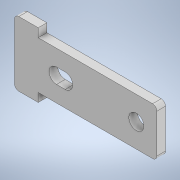
# Autodesk Inventor part: Крепеж
Saved by Autodesk Inventor 2021 (Build 250183000, 183)
## iProperties
Created: 2022-07-08
Part Number: Крепеж
Material: Типовые
Document SubType Name: Modeling
Designer: zvi20
Density: 1 g/cm^3
Appearance: По умолчанию
Author: zvi20
Autodesk Inventor part; units mm, degrees
ref_plane "YZ Plane" through (0, 0, 0) normal (1, 0, 0) x (0, 1, 0)
ref_plane "XZ Plane" through (0, 0, 0) normal (0, 1, 0) x (-1, 0, 0)
ref_plane "XY Plane" through (0, 0, 0) normal (0, 0, 1) x (1, 0, 0)
sketch "Эскиз1" plane through (0, 0, 0) normal (0, 0, 1) x (1, 0, 0)
  line L0 (-4.6809, -0.7904) -> (-4.6809, 1.2096)
  line L1 (-4.6809, -13.7904) -> (-4.6809, -11.7904)
  line L2 (-4.6809, 1.2096) -> (-9.1809, 1.2096)
  line L3 (-10.1809, 0.2096) -> (-10.1809, -12.7904)
  line L4 (-9.1809, -13.7904) -> (-4.6809, -13.7904)
  arc A0 (-10.1809, -12.7904) -> (-9.1809, -13.7904) centre (-9.1809, -12.7904) ccw
  arc A1 (-9.1809, 1.2096) -> (-10.1809, 0.2096) centre (-9.1809, 0.2096) ccw
  line L5 (22.8191, -1.7904) -> (22.8191, -10.7904)
  line L6 (21.8191, -11.7904) -> (-4.6809, -11.7904)
  line L7 (-4.6809, -0.7904) -> (21.8191, -0.7904)
  arc A2 (22.8191, -1.7904) -> (21.8191, -0.7904) centre (21.8191, -1.7904) ccw
  arc A3 (21.8191, -11.7904) -> (22.8191, -10.7904) centre (21.8191, -10.7904) ccw
  arc A4 (-0.4309, -4.5404) -> (-0.4309, -8.0404) centre (-0.4309, -6.2904) ccw
  arc A5 (1.5691, -8.0404) -> (1.5691, -4.5404) centre (1.5691, -6.2904) ccw
  line L8 (-0.4309, -4.5404) -> (1.5691, -4.5404)
  line L9 (-0.4309, -8.0404) -> (1.5691, -8.0404)
  circle A6 centre (18.0691, -6.2904) radius 1.75
  point P0 (0, 0)
  point P1 (-10.1809, 1.2096)
  point P2 (-10.1809, -13.7904)
  point P3 (22.8191, -0.7904)
  point P4 (22.8191, -11.7904)
  constraints: 20 end point, 12 point on circle, 10 point on line, 10 tangent, 7 centre point, 2 equal radius, 2 perpendicular, 1 horizontal, 1 parallel
extrude "Выдавливание2" add sketch "Эскиз1" along normal blind 2
